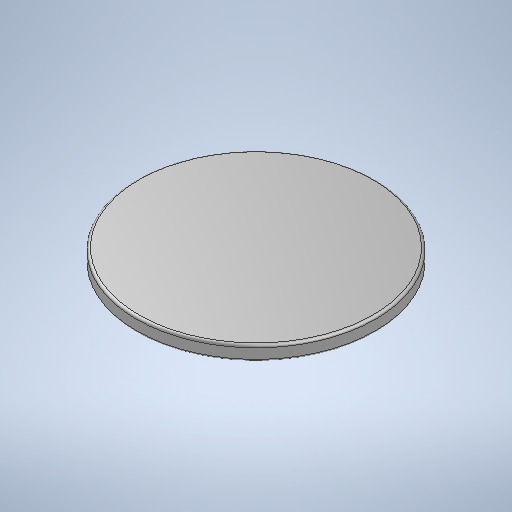
# Autodesk Inventor part: Base Disk Model
Saved by Autodesk Inventor 2025.1 (Build 291241000, 241)
## iProperties
Created: 2025-10-25
Part Number: Base Disk Model
Material: Generic
Document SubType Name: Modeling
Designer: benja
Density: 1 g/cm^3
Appearance: Anodized - Light Gray
Author: benja
Autodesk Inventor part; units mm, degrees
ref_plane "YZ Plane" through (0, 0, 0) normal (1, 0, 0) x (0, 1, 0)
ref_plane "XZ Plane" through (0, 0, 0) normal (0, 1, 0) x (-1, 0, 0)
ref_plane "XY Plane" through (0, 0, 0) normal (0, 0, 1) x (1, 0, 0)
sketch "Sketch1" plane through (0, 0, 0) normal (0, 1, 0) x (-1, 0, 0)
  circle A0 centre (0, 0) radius 152.4
  line L0 (69.2907, -40.005) -> (62.6916, -36.195)
  line L1 (-62.6916, -36.195) -> (-69.2907, -40.005)
  line L2 (0, 72.39) -> (0, 80.01)
  line L3 (65.9911, -38.1) -> (15.1911, -126.0882)
  line L4 (65.9911, -38.1) -> (116.7911, 49.8882)
  line L5 (15.1911, -126.0882) -> (116.7911, 49.8882) construction
  line L6 (11.8916, -124.1832) -> (113.4916, 51.7932)
  line L7 (120.0907, 47.9832) -> (18.4907, -127.9932)
  arc A1 (11.8916, -124.1832) -> (18.4907, -127.9932) centre (15.1911, -126.0882) ccw
  arc A2 (120.0907, 47.9832) -> (113.4916, 51.7932) centre (116.7911, 49.8882) ccw
  circle A3 centre (0, -132.08) radius 9.017
  circle A4 centre (114.3846, 66.04) radius 9.017
  circle A5 centre (-114.3846, 66.04) radius 9.017
  line L8 (-101.6, 80.01) -> (101.6, 80.01)
  line L9 (101.6, 72.39) -> (-101.6, 72.39)
  arc A6 (101.6, 72.39) -> (101.6, 80.01) centre (101.6, 76.2) ccw
  arc A7 (-101.6, 80.01) -> (-101.6, 72.39) centre (-101.6, 76.2) ccw
  line L10 (-18.4907, -127.9932) -> (-120.0907, 47.9832)
  line L11 (-113.4916, 51.7932) -> (-11.8916, -124.1832)
  arc A8 (-113.4916, 51.7932) -> (-120.0907, 47.9832) centre (-116.7911, 49.8882) ccw
  arc A9 (-18.4907, -127.9932) -> (-11.8916, -124.1832) centre (-15.1911, -126.0882) ccw
  circle A10 centre (0, 0) radius 9.017
  dimension "d4" = 304.8
  dimension "d5" = 101.6
  dimension "d6" = 101.6
  dimension "d8" = 18.034
  dimension "d11" = 360
  dimension "d15" = 360
  dimension "d17" = 18.034
  constraints: 26 end point, 12 point on circle, 11 centre point, 4 tangent, 2 coincident, 2 midpoint, 1 parallel, 38 other
  measures "d4" diameter of A0
  measures "d5" distance of L3.start L3.end
  measures "d6" distance of L3.start L4.end
  measures "d8" diameter of A3
  measures "d17" diameter of A10
extrude "Extrusion1" add sketch "Sketch1" against normal blind 19.05 contours A0 | L7 A1 L6 L0 | L0 L6 A2 L7 | L11 A9 L10 L1 | L1 L10 A8 L11 | L9 A7 L8 L2 | L2 L8 A6 L9 | A3 | A4 | A5 | A10
fillet "Fillet1" radius 3.175 2 edges at (152.4, 0, 0) (152.4, -19.05, 0)
body "Solid1"
